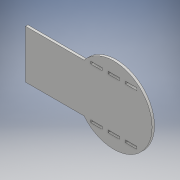
# Autodesk Inventor part: base3
Saved by Autodesk Inventor 2018 (Build 220112000, 112)
## iProperties
Created: 2020-03-10
Part Number: base3
Material: Genérico
Document SubType Name: Modeling
Designer: sala.ceri
Density: 1 g/cm^3
Appearance: Valor por defecto
Author: sala.ceri
Autodesk Inventor part; units mm, degrees
ref_plane "YZ Plane" through (0, 0, 0) normal (1, 0, 0) x (0, 1, 0)
ref_plane "XZ Plane" through (0, 0, 0) normal (0, 1, 0) x (-1, 0, 0)
ref_plane "XY Plane" through (0, 0, 0) normal (0, 0, 1) x (1, 0, 0)
sketch "Boceto1" plane through (0, 0, 0) normal (0, 1, 0) x (-1, 0, 0)
  circle A0 centre (28.5, 0) radius 1.5
  circle A1 centre (28.5, -8) radius 1.5
  circle A2 centre (28.5, 8) radius 1.5
  circle A3 centre (36.5, 0) radius 1.5
  circle A4 centre (20.5, 0) radius 1.5
  circle A5 centre (28.5, 0) radius 47.5
  line L0 (57, 33) -> (43, 33)
  line L1 (43, 33) -> (43, 30)
  line L2 (35.5, 30) -> (35.5, 33)
  line L3 (35.5, 33) -> (21.5, 33)
  line L4 (21.5, 33) -> (21.5, 30)
  line L5 (14, 30) -> (14, 33)
  line L6 (14, 33) -> (0, 33)
  line L7 (43, 30) -> (57, 30)
  line L8 (21.5, 30) -> (35.5, 30)
  line L9 (14, 30) -> (0, 30)
  line L10 (0, 30) -> (0, 33)
  line L11 (57, 33) -> (57, 30)
  line L12 (35.5, -30) -> (35.5, -33)
  line L13 (21.5, -30) -> (35.5, -30)
  line L14 (35.5, -33) -> (21.5, -33)
  line L15 (21.5, -33) -> (21.5, -30)
  line L16 (57, -33) -> (43, -33)
  line L17 (43, -33) -> (43, -30)
  line L18 (43, -30) -> (57, -30)
  line L19 (14, -30) -> (14, -33)
  line L20 (14, -30) -> (0, -30)
  line L21 (14, -33) -> (0, -33)
  line L22 (0, -30) -> (0, -33)
  line L23 (57, -33) -> (57, -30)
  constraints: 48 end point, 10 point on line, 6 centre point, 1 coincident, 1 vertical
extrude "Extrusión1" add sketch "Boceto1" along normal blind 3
sketch "Boceto2" plane through (-28.5, 0, 0) normal (0, -1, 0) x (1, 0, 0)
  circle A0 centre (0, 0) radius 3.5
  point P0 (28.5, 0)
  dimension "d23" = 7
  constraints: 1 centre point
  measures "d23" diameter of A0
extrude "Extrusión2" cut sketch "Boceto2" against normal blind 10
sketch "Boceto3" plane through (-28.5, 0, 0) normal (0, -1, 0) x (1, 0, 0)
  circle A0 centre (0, 0) radius 4.5
  point P0 (28.5, 0)
  dimension "d26" = 9
  constraints: 1 centre point
  measures "d26" diameter of A0
extrude "Extrusión3" cut sketch "Boceto3" against normal blind 10
sketch "Boceto4" plane through (-28.5, 0, 0) normal (0, -1, 0) x (1, 0, 0)
  arc A0 (-36.5, 30) -> (-36.5, -30) centre (0, 0) ccw
  line L0 (-28.5, 30) -> (-28.5, 33) projected
  line L1 (-36.5, 30) -> (-109.5, 30)
  line L2 (-109.5, 30) -> (-109.5, -30)
  line L3 (-28.5, -33) -> (-28.5, -30) projected
  line L4 (-109.5, -30) -> (-36.5, -30)
  constraints: 6 end point, 2 perpendicular, 2 point on circle, 1 centre point, 1 coincident
extrude "Extrusión4" add sketch "Boceto4" against normal blind 3
sketch "Boceto5" plane through (0, 3, 0) normal (0, 1, 0) x (1, 0, 0)
  line L0 (-11.1092, 17.1983) -> (-42.6801, 17.1983)
  line L1 (-42.6801, 17.1983) -> (-42.6801, -13.2583)
  line L2 (-42.6801, -13.2583) -> (-11.1092, -13.2583)
  line L3 (-11.1092, -13.2583) -> (-11.1092, 17.1983)
  point P0 (0, 0)
  constraints: 8 end point, 2 parallel, 1 horizontal, 1 perpendicular
extrude "Extrusión5" add sketch "Boceto5" against normal blind 3
